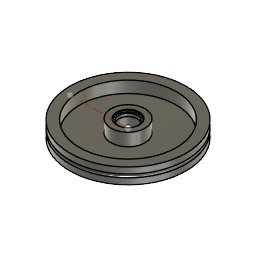
Guide_Pulley_120mm (Autodesk Fusion 360 design; units mm, degrees)
part number: 2026-08-12-12-54-22-728
Autodesk Fusion 360 part; units mm, degrees
sketch "草图1" plane through (0, 0, 0) normal (0, 0, 1) x (1, 0, 0)
  circle A0 centre (0, 0) radius 60
  circle A1 centre (0, 0) radius 11.25
  dimension "d19" = 120
  dimension "d20" = 22.5
  constraint coincident A0.centre A1.centre
  measures "d19" diameter of A0
  measures "d20" diameter of A1
extrude "拉伸1" add sketch "草图1" along normal blind 4 makes body 1
sketch "草图2" plane through (0, 0, 4) normal (0, 0, 1) x (-1, 0, 0)
  circle A0 centre (0, 0) radius 11.25
  circle A1 centre (0, 0) radius 60
  circle A2 centre (0, 0) radius 60
  circle A3 centre (0, 0) radius 50
  dimension "d23" = 100
  constraint concentric A2 A3
  measures "d23" diameter of A3
extrude "拉伸2" add sketch "草图2" along normal blind 12 contours A1 A2 bodies 1
sketch "草图3" plane through (0, 0, 4) normal (0, 0, 1) x (-1, 0, 0)
  circle A0 centre (0, 0) radius 50
  circle A1 centre (0, 0) radius 11.25
  circle A2 centre (0, 0) radius 11.25
  circle A3 centre (0, 0) radius 17.5
  dimension "d26" = 35
  constraint concentric A2 A3
  measures "d26" diameter of A3
extrude "拉伸3" add sketch "草图3" along normal blind 13 contours A3 bodies 1
sketch "草图4" plane through (0, 0, 0) normal (0, 1, 0) x (1, 0, 0)
  line L0 (0, 0) -> (0, -8) construction
  dimension "d29" = 8
  constraint coincident L0.start origin
  constraint vertical L0
  measures "d29" distance of L0.start L0.end
sketch "草图5" plane through (0, 0, 0) normal (0, 1, 0) x (1, 0, 0)
  line L0 (0, -8) -> (-59.9, -8) construction
  dimension "d30" = 59.9
  constraint horizontal L0
  measures "d30" distance of L0.start L0.end
sketch "草图6" plane through (0, 0, 0) normal (0, 1, 0) x (1, 0, 0)
  circle A0 centre (-60, -8) radius 1.7
  dimension "d31" = 3.4
  measures "d31" diameter of A0
revolve "旋转1" cut sketch "草图6" angle 360 about axis through (0, 0, 0) along (0, 0, 1) bodies 1
sketch "草图8" plane through (0, 0, 0) normal (0, 0, -1) x (1, 0, 0)
  circle A0 centre (0, 0) radius 11.25
  circle A1 centre (0, 0) radius 60
  circle A2 centre (0, 0) radius 9.5
  dimension "d36" = 19
  constraint coincident A0.centre A1.centre
  measures "d36" diameter of A2
extrude "拉伸4" add sketch "草图8" against normal blind 15 separate body contours A0 makes body 2
extrude "拉伸5" cut 1 faces at (10.5894, 1.0309, 0) along direction (0, 0, 1) blind 12 on bodies 2 bodies 2
chamfer "倒角1" distance 0.4 angle 45 2 edges at (10.4887, -4.0682, 17) (-10.4887, 4.0682, 0) on bodies 1
equation "Pulley_Outer_Diameter = 120 mm" comment "大导向轮外径"
equation "Pulley_Total_Height = 16 mm" comment "大导向轮总高度"
equation "Rim_Inner_Diameter = 100 mm" comment "外圈轮缘内径"
equation "Hub_Outer_Diameter = 32 mm" comment "中央轮毂外径"
equation "Web_Thickness = 4 mm" comment "底部连续腹板厚度"
equation "Bearing_OD = 22 mm" comment "608轴承外径"
equation "Bearing_ID = 8 mm" comment "608轴承内径"
equation "Bearing_Width = 7 mm" comment "单个608轴承宽度"
equation "Bearing_Seat_Diameter = 22.2 mm" comment "V1轴承座孔CAD起始值；打印测试后按0.05-0.1 mm调整"
equation "Bearing_LeadIn_Chamfer = 0.4 mm" comment "上下轴承孔入口导入倒角"
equation "Catheter_Diameter = 2.4 mm" comment "实际弹簧导管外径"
equation "Groove_Width = 3.4 mm" comment "外圆周导管槽切除圆直径/名义槽宽"
equation "Groove_Depth = 1.8 mm" comment "导管槽相对原始外圆的最大径向深度"
equation "Groove_Radius = Groove_Width / 2" comment "导管槽切除圆半径"
equation "Groove_Center_Inset = Groove_Depth - Groove_Radius" comment "槽圆心相对原始外圆向内偏置"
equation "Groove_Center_Radius = Pulley_Outer_Diameter / 2 - Groove_Center_Inset" comment "从轮中心Z轴到槽截面圆心的径向距离"
equation "Groove_Center_Height = Pulley_Total_Height / 2" comment "槽中心距轮子底面的高度"
equation "Groove_Entry_Fillet = 0.3 mm" comment "导管槽上下入口边缘小圆角；若求解失败V1可删除"
equation "d19 = Pulley_Outer_Diameter"
equation "d20 = Bearing_Seat_Diameter + 0.3 mm"
equation "d21 = Web_Thickness"
equation "d23 = Rim_Inner_Diameter"
equation "d24 = Pulley_Total_Height - Web_Thickness"
equation "d26 = Hub_Outer_Diameter + 3 mm"
equation "d29 = Groove_Center_Height"
equation "d30 = Groove_Center_Radius"
equation "d31 = Groove_Width"
equation "d33 = Bearing_LeadIn_Chamfer"
